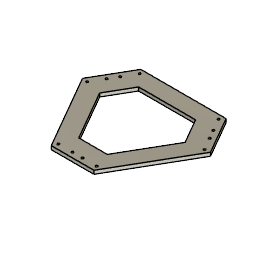
Stewart's Stationary Base (Autodesk Fusion 360 design; units mm, degrees)
Autodesk Fusion 360 part; units mm, degrees
sketch "Sketch2" plane through (0, 0, 0) normal (0, 0, 1) x (1, 0, 0)
  line L0 (0, 0) -> (-120, 0)
  line L1 (-120, 0) -> (-150, -51.9615)
  line L2 (0, 0) -> (30, -51.9615)
  line L3 (30, -51.9615) -> (-30, -155.8846)
  line L4 (-30, -155.8846) -> (-90, -155.8846)
  line L5 (-90, -155.8846) -> (-150, -51.9615)
  circle A0 centre (-33, -148.8846) radius 1.5
  circle A1 centre (-53, -148.8846) radius 1.5
  circle A2 centre (-87, -148.8846) radius 1.5
  circle A3 centre (-67, -148.8846) radius 1.5
  circle A4 centre (-142.4378, -52.8634) radius 1.5
  line L6 (-150, -51.9615) -> (-139.3427, -58.1145) construction
  line L7 (-109.3484, -6.1497) -> (-120, 0) construction
  circle A5 centre (-132.4378, -35.5429) radius 1.5
  circle A6 centre (-115.4378, -6.0981) radius 1.5
  circle A7 centre (-125.4378, -23.4186) radius 1.5
  line L8 (30, -51.9615) -> (24.7639, -54.9846) construction
  line L9 (0, 0) -> (-6.3914, -3.69) construction
  circle A8 centre (-4.5622, -6.0981) radius 1.5
  circle A9 centre (5.4378, -23.4186) radius 1.5
  circle A10 centre (22.4378, -52.8634) radius 1.5
  circle A11 centre (12.4378, -35.5429) radius 1.5
  line L10 (-135, -25.9808) -> (0, -103.923) construction
  line L11 (15, -25.9808) -> (-120, -103.923) construction
  line L12 (-60, -155.8846) -> (-60, 0) construction
  circle A12 centre (-60, -69.282) radius 1.5
  line L13 (-100, -23.094) -> (-20, -23.094)
  line L14 (-20, -23.094) -> (0, -57.735)
  line L15 (0, -57.735) -> (-40, -127.0171)
  line L16 (-40, -127.0171) -> (-80, -127.0171)
  line L17 (-80, -127.0171) -> (-120, -57.735)
  line L18 (-120, -57.735) -> (-100, -23.094)
  dimension "d1" = 120
  dimension "d2" = 60
  dimension "d8" = 60
  dimension "d9" = 120
  dimension "d10" = 60
  dimension "d13" = 120
  dimension "d14" = 3
  dimension "d15" = 7
  dimension "d16" = 3
  dimension "d17" = 3
  dimension "d18" = 20
  dimension "d19" = 7
  dimension "d20" = 3
  dimension "d21" = 3
  dimension "d22" = 7
  dimension "d23" = 3
  dimension "d24" = 7
  dimension "d25" = 20
  dimension "d26" = 3
  dimension "d27" = 3
  dimension "d28" = 7
  dimension "d29" = 3
  dimension "d30" = 20
  dimension "d31" = 7
  dimension "d32" = 3
  dimension "d33" = 3
  dimension "d34" = 3
  dimension "d35" = 7
  dimension "d36" = 20
  dimension "d37" = 7
  dimension "d38" = 3
  dimension "d39" = 3
  dimension "d40" = 7
  dimension "d41" = 3
  dimension "d42" = 3
  dimension "d43" = 3
  dimension "d44" = 7
  dimension "d45" = 20
  dimension "d46" = 3
  dimension "d47" = 7
  dimension "d48" = 7
  dimension "d49" = 20
  dimension "d50" = 3
  dimension "d51" = 40
  dimension "d52" = 80
  dimension "d53" = 40
  dimension "d54" = 80
  dimension "d56" = 20
  dimension "d57" = 40
  constraint coincident L0.start L2.start
  constraint horizontal L0
  constraint perpendicular L1 L6
  constraint perpendicular L1 L7
  constraint perpendicular L2 L8
  constraint perpendicular L2 L9
  constraint parallel L1 L3
  constraint parallel L2 L5
  constraint parallel L0 L4
  constraint midpoint L1 L10.start
  constraint midpoint L3 L10.end
  constraint midpoint L2 L11.start
  constraint midpoint L5 L11.end
  constraint midpoint L4 L12.start
  constraint perpendicular L4 L12
  constraint midpoint L0 L12.end
  constraint coincident L12 A12.centre
  constraint coincident L11 A12.centre
  constraint perpendicular L12 L13
  constraint perpendicular L11 L14
  constraint perpendicular L10 L15
  constraint perpendicular L12 L16
  constraint perpendicular L11 L17
  constraint perpendicular L10 L18
  measures "d1" distance of L0.start L0.end
  measures "d2" distance of L0.end L1.end
  measures "d8" distance of L0.start L2.end
  measures "d9" distance of L2.end L3.end
  measures "d10" distance of L3.end L4.end
  measures "d13" distance of L1.end L4.end
  measures "d14" diameter of A0
  measures "d15" distance of L4 A0.centre
  measures "d16" horizontal distance of L3.end A0.centre
  measures "d17" diameter of A1
  measures "d18" horizontal distance of A0.centre A1.centre
  measures "d19" distance of L4 A1.centre
  measures "d20" diameter of A2
  measures "d21" horizontal distance of L4.end A2.centre
  measures "d22" distance of L4 A2.centre
  measures "d23" diameter of A3
  measures "d24" distance of L4 A3.centre
  measures "d25" distance of A2.centre A3.centre
  measures "d26" diameter of A4
  measures "d27" distance of A4.centre L6
  measures "d28" distance of L1 A4.centre
  measures "d29" diameter of A5
  measures "d30" distance of A4.centre A5.centre
  measures "d31" distance of L1 A5.centre
  measures "d32" diameter of A6
  measures "d33" distance of L7 A6.centre
  measures "d34" diameter of A7
  measures "d35" distance of L1 A6.centre
  measures "d36" distance of A6.centre A7.centre
  measures "d37" distance of L1 A7.centre
  measures "d38" diameter of A8
  measures "d39" distance of L9 A8.centre
  measures "d40" distance of L2 A8.centre
  measures "d41" diameter of A9
  measures "d42" diameter of A10
  measures "d43" diameter of A11
  measures "d44" distance of L2 A9.centre
  measures "d45" distance of A8.centre A9.centre
  measures "d46" distance of L8 A10.centre
  measures "d47" distance of L2 A10.centre
  measures "d48" distance of L2 A11.centre
  measures "d49" distance of A10.centre A11.centre
  measures "d50" diameter of A12
  measures "d51" distance of L13.end L14.end
  measures "d52" distance of L14.end L15.end
  measures "d53" distance of L15.end L16.end
  measures "d54" distance of L16.end L17.end
  measures "d56" distance of L11 L13.end
  measures "d57" distance of L12 L13.end
extrude "Extrude1" add sketch "Sketch2" along normal blind 5 contours L0 L1 L2 L3 L4 L5
named bodies: "Base Plate"
